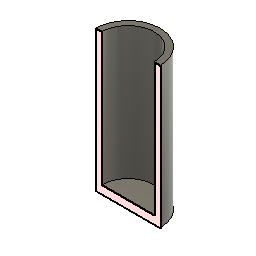
tubeToolHolder04 (Autodesk Fusion 360 design; units mm, degrees)
Autodesk Fusion 360 part; units mm, degrees
sketch "Sketch1" plane through (0, 0, 0) normal (0, 1, 0) x (1, 0, 0)
  circle A0 centre (0, 0) radius 16
  circle A1 centre (0, 0) radius 13
  dimension "d1" = 32
  dimension "d7" = 3
  constraint coincident A0.centre A1.centre
  measures "d1" diameter of A0
  measures "d7" distance of A0 A1
extrude "Extrude1" add sketch "Sketch1" along normal blind 70 makes body 1
extrude "Extrude2" add sketch "Sketch1" along normal blind 4 contours A1 bodies 1
copy_body "Body->Comp1" bodies 1 removing the originals makes body 2 in component "tubeToolHolder04"
component "tubeToolHolder04" placed x (1, 0, 0) y (0, 1, 0) z (0, 0, 1) at (0, 0, 0)
